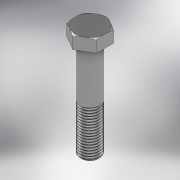
# Autodesk Inventor part: Part16 Real Bolt Thread
Saved by Autodesk Inventor 2022.2 (Build 262287010, 287A)
## iProperties
Created: 2022-12-19
Part Number: Part16 Real Bolt Thread
Material: Steel
Document SubType Name: Modeling
Designer: User
Mass: 527.789 g
Surface Area: 152.44 cm^2
Volume: 67.2343 cm^3
Density: 7.85 g/cm^3
Appearance: Semi-Polished
Author: User
Autodesk Inventor part; units mm, degrees
ref_plane "YZ Plane" through (0, 0, 0) normal (1, 0, 0) x (0, 1, 0)
ref_plane "XZ Plane" through (0, 0, 0) normal (0, 1, 0) x (-1, 0, 0)
ref_plane "XY Plane" through (0, 0, 0) normal (0, 0, 1) x (1, 0, 0)
sketch "Sketch1" plane through (0, 0, 0) normal (0, 1, 0) x (-1, 0, 0)
  line L0 (127.8939, 73.8396) -> (127.8939, -73.8396)
  line L1 (127.8939, -73.8396) -> (0, -147.6791)
  line L2 (0, -147.6791) -> (-127.8939, -73.8396)
  line L3 (-127.8939, -73.8396) -> (-127.8939, 73.8396)
  line L4 (-127.8939, 73.8396) -> (0, 147.6791)
  line L5 (0, 147.6791) -> (127.8939, 73.8396)
  line L6 (-18, 10.3923) -> (0, 20.7846)
  line L7 (0, 20.7846) -> (18, 10.3923)
  line L8 (18, 10.3923) -> (18, -10.3923)
  line L9 (18, -10.3923) -> (0, -20.7846)
  line L10 (0, -20.7846) -> (-18, -10.3923)
  line L11 (-18, -10.3923) -> (-18, 10.3923)
  point P0 (0, 0)
  point P1 (0, 0)
  point P2 (0, 0)
  dimension "d1" = 36
  constraints: 24 end point, 2 coincident, 2 vertical, 26 other
  measures "d1" distance between parallel lines of L11 L8
extrude "Extrusion1" add sketch "Sketch1" along normal blind 15 contours L6 L7 L8 L9 L10 L11
sketch "Sketch2" plane through (0, 0, 0) normal (1, 0, 0) x (0, 1, 0)
  line L0 (0, -20.7846) -> (15, -20.7846) construction
  line L1 (15, -20.7846) -> (13.3923, -20.7846)
  line L2 (13.3923, -20.7846) -> (15, -18)
  line L3 (15, -18) -> (15, -20.7846)
  line L4 (-3, 0) -> (18, 0) projected
  point P0 (0, 0)
  dimension "d4" = 60
  dimension "d5" = 36
  constraints: 6 end point, 1 point on line, 1 vertical
  measures "d4" angle of L2 L0
  measures "d5" diameter of L2.end L4
revolve "Revolution1" cut sketch "Sketch2" angle 360 about axis through (0, -10, 0) along (0, 1, 0)
sketch "Sketch3" plane through (0, 0, 0) normal (0, 0, 1) x (1, 0, 0)
  line L0 (0, 0) -> (12, 0)
  line L1 (12, 0) -> (12, -120)
  line L2 (12, -120) -> (0, -120)
  line L3 (0, -120) -> (0, 0)
  dimension "d7" = 120
  dimension "d8" = 24
  constraints: 8 end point, 2 parallel, 1 horizontal, 1 perpendicular
  measures "d7" distance of L0.end L1.end
  measures "d8" diameter of L1 L3
revolve "Revolution2" add sketch "Sketch3" angle 360 about axis through (0, -120, 0) along (0, 1, 0)
fillet "Fillet1" radius 0.8 1 edges at (-12, 0, 0)
chamfer "Chamfer1" distance 2 angle 45 1 edges at (-12, -120, 0)
sketch "Sketch4" plane through (0, 0, 0) normal (0, 0, 1) x (1, 0, 0)
  line L0 (0, -147) -> (0, 42) projected
  line L1 (12, -0.8) -> (12, -118) construction
  line L2 (12, -62.6874) -> (10.376, -63.625)
  line L3 (10.376, -63.625) -> (10.376, -64.375) construction
  line L4 (10.376, -64.375) -> (12, -65.3126)
  line L5 (12, -62.6874) -> (12, -65.3126)
  line L6 (11.0255, -63.25) -> (11.0255, -64.75) construction
  arc A0 (10.376, -63.625) -> (10.376, -64.375) centre (10.5925, -64) ccw
  line L7 (10, -120) -> (-10, -120) projected
  point P0 (0, 0)
  point P1 (10.376, -64)
  dimension "d16" = 60
  dimension "d17" = 22.051
  dimension "d18" = 1.5
  dimension "d19" = 20.752
  dimension "d20" = 56
  constraints: 10 end point, 4 point on line, 3 vertical, 2 point on circle, 2 tangent, 1 centre point, 1 equal length, 1 midpoint
  measures "d16" angle of L4 L2
  measures "d17" diameter of L6 L0
  measures "d18" distance of L6.start L6.end
  measures "d19" diameter of point (10.376, -64) L0
  measures "d20" distance from line of L7 point (10.376, -64)
coil "Coil1" sketch "Sketch4" operation cut axis through (0, -10, 0) along (0, -1, 0) pitch 3 turns 20 hand right
sketch "Sketch5" plane through (10.5925, -64, 0) normal (0, 0, 1) x (1, 0, 0)
  line L0 (1.4075, 1.3126) -> (-0.2165, 0.375) projected
  arc A0 (-0.2165, 0.375) -> (-0.2165, -0.375) centre (0, 0) ccw projected
  line L1 (-0.2165, -0.375) -> (1.4075, -1.3126) projected
  line L2 (1.4075, 1.3126) -> (1.4075, -1.3126) projected
  point P0 (-10.5925, 64)
extrude "Extrusion2" cut sketch "Sketch5" against normal through all
equation "\"d5\" = d1"
body "Solid1"
